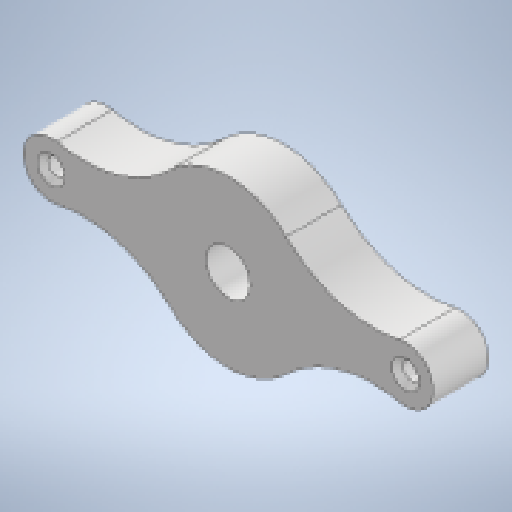
# Autodesk Inventor part: Brida_Rodamiento
Saved by Autodesk Inventor 2024 (Build 280153000, 153)
## iProperties
Created: 2024-07-16
Part Number: Brida_Rodamiento
Material: Genérico
Document SubType Name: Modeling
Designer: sergi
Density: 1 g/cm^3
Appearance: Valor por defecto
Author: sergi
Autodesk Inventor part; units mm, degrees
ref_plane "YZ Plane" through (0, 0, 0) normal (1, 0, 0) x (0, 1, 0)
ref_plane "XZ Plane" through (0, 0, 0) normal (0, 1, 0) x (-1, 0, 0)
ref_plane "XY Plane" through (0, 0, 0) normal (0, 0, 1) x (1, 0, 0)
sketch "Boceto1" plane through (0, 0, 0) normal (0, 0, 1) x (1, 0, 0)
  circle A0 centre (0, 0) radius 8.25 projected
  arc A1 (-36.7643, -25.9497) -> (36.7643, -25.9497) centre (0, 0) ccw projected
  arc A2 (-35.5756, -20.5396) -> (-36.7643, -25.9497) centre (-33.7006, -23.7872) ccw projected
  line L0 (-35.5756, -20.5396) -> (-15.9099, -9.1856) projected
  arc A3 (-11.2279, -9.9465) -> (-15.9099, -9.1856) centre (-14.0349, -12.4332) ccw projected
  arc A4 (-11.2279, -9.9465) -> (11.2279, -9.9465) centre (0, 0) ccw projected
  arc A5 (15.9099, -9.1856) -> (11.2279, -9.9465) centre (14.0349, -12.4332) ccw projected
  line L1 (15.9099, -9.1856) -> (35.5756, -20.5396) projected
  arc A6 (36.7643, -25.9497) -> (35.5756, -20.5396) centre (33.7006, -23.7872) ccw projected
  line L2 (98, -98) -> (98, 98) projected
  line L3 (98, 98) -> (-98, 98) projected
  line L4 (-98, 98) -> (-98, -98) projected
  line L5 (-98, -98) -> (98, -98) projected
  circle A7 centre (0, 0) radius 4 projected
  line L6 (21.4655, -12.3931) -> (15.9099, -9.1856) projected
  arc A8 (15.9099, -9.1856) -> (11.2279, -9.9465) centre (14.0349, -12.4332) ccw projected
  arc A9 (-11.2279, -9.9465) -> (11.2279, -9.9465) centre (0, 0) ccw projected
  arc A10 (-11.2279, -9.9465) -> (-15.9099, -9.1856) centre (-14.0349, -12.4332) ccw projected
  line L7 (-15.9099, -9.1856) -> (-21.4655, -12.3931) projected
  line L8 (0, 0) -> (-32, 0) construction
  line L9 (0, 0) -> (32, 0) construction
  circle A11 centre (-32, 0) radius 1.5
  circle A12 centre (0, 0) radius 4
  circle A13 centre (-32, 0) radius 5
  circle A14 centre (0, 0) radius 15
  circle A15 centre (26.1563, -26.8719) radius 22.5
  circle A16 centre (-26.1562, -26.8719) radius 22.5
  circle A17 centre (-26.1562, 26.8719) radius 22.5
  circle A18 centre (26.1563, 26.8719) radius 22.5
  line L10 (0, 0) -> (32, 0) construction
  circle A19 centre (32, 0) radius 5
  circle A20 centre (32, 0) radius 1.5
  line L11 (21.4655, -12.3931) -> (21.4655, 21.4655) projected
  line L12 (-21.4655, 21.4655) -> (-21.4655, -12.3931) projected
  line L13 (21.4655, 21.4655) -> (-21.4655, 21.4655) projected
  point P0 (0, 0)
  point P1 (21.8181, -12.5967)
  point P2 (-21.8181, -12.5967)
  point P3 (-11.6313, -9.4678)
  point P4 (-10.4625, 10.7488)
  point P5 (-30.9375, 4.8858)
  point P6 (-30.9375, -4.8858)
  point P7 (-12.4296, -9.0441)
  point P8 (12.4296, -9.0441)
  point P9 (10.4625, 10.7488)
  point P10 (-11.1152, -43.6056)
  point P11 (11.1152, -43.6056)
  point P12 (-10.4625, -10.7488)
  point P13 (10.4625, -10.7488)
  point P14 (11.2279, -9.9465)
  point P15 (11.2279, -9.9465)
  point P16 (30.9375, -4.8858)
  point P17 (30.9375, 4.8858)
  dimension "d3" = 180
  dimension "d4" = 3
  dimension "d16" = 10
  dimension "d18" = 32
  dimension "d19" = 30
  dimension "empalme" = 45
  dimension "d22" = 45
  dimension "d23" = 45
  dimension "d24" = 45
  dimension "d27" = 32
  dimension "d28" = 10
  dimension "d29" = 3
  constraints: 10 centre point, 8 tangent, 6 coincident, 6 end point, 2 horizontal, 1 collinear, 1 concentric, 1 point on line
  measures "d3" angle of L8 L9
  measures "d4" diameter of A11
  measures "d16" diameter of A13
  measures "d18" distance of L8.start L8.end
  measures "d19" diameter of A14
  measures "empalme" diameter of A15
  measures "d22" diameter of A16
  measures "d23" diameter of A17
  measures "d24" diameter of A18
  measures "d27" distance of L10.start L10.end
  measures "d28" diameter of A19
  measures "d29" diameter of A20
extrude "Extrusión1" add sketch "Boceto1" along normal blind 10 contours A0 | A13 | A13 A17 L12 A16 | A4 A14 | A4 A5 A15 | L12 A17 A14 A3 A16 | A16 A3 A4 | A14 A18 L11 A15 A5 | A15 L11 A18 A19 | A19
sketch "Boceto2" plane through (0, 0, 0) normal (0, 0, -1) x (-1, 0, 0)
  circle A0 centre (0, 0) radius 8.25 projected
  point P0 (0, 0)
extrude "Extrusión2" cut sketch "Boceto2" against normal blind 3
sketch "Boceto3" plane through (0, 0, 3) normal (0, 0, -1) x (-1, 0, 0)
  circle A0 centre (0, 0) radius 5.25 projected
  point P0 (0, 0)
extrude "Extrusión3" cut sketch "Boceto3" against normal blind 0.5
chamfer "Chaflán1" distance 1 angle 45 2 edges at (30.5, 0, 10) (-33.5, 0, 10) measured on face at (-11.2475, 0, 10)
equation "\"d22\" = empalme"
equation "\"d23\" = empalme"
equation "\"d24\" = empalme"
